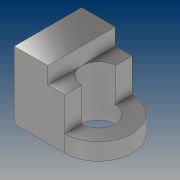
# Autodesk Inventor part: 34
Saved by Autodesk Inventor 2020.2 (Build 242310000, 310)
## iProperties
Created: 2020-09-17
Part Number: 34
Material: 鋼、碳鋼
Document SubType Name: Modeling
Designer: user
Density: 7.85 g/cm^3
Appearance: 半拋光
Mass: 345.4 g
Surface Area: 95.1327 cm^2
Volume: 44 cm^3
Author: user
Autodesk Inventor part; units mm, degrees
ref_plane "YZ Plane" through (0, 0, 0) normal (1, 0, 0) x (0, 1, 0)
ref_plane "XZ Plane" through (0, 0, 0) normal (0, 1, 0) x (-1, 0, 0)
ref_plane "XY Plane" through (0, 0, 0) normal (0, 0, 1) x (1, 0, 0)
sketch "草圖1" plane through (0, 0, 0) normal (0, 1, 0) x (-1, 0, 0)
  circle A0 centre (0, 0) radius 20
  line L0 (0, -20) -> (30, -20)
  line L1 (30, -20) -> (30, 20)
  line L2 (30, 20) -> (0, 20)
  line L3 (0, 20) -> (0, -20)
  point P0 (0, 20)
  dimension "d0" = 40
  dimension "d1" = 30
  constraints: 8 end point, 3 horizontal, 2 parallel, 1 coincident, 1 perpendicular, 3 other
  measures "d1" distance of L1.end L2.end
extrude "擠出1" add sketch "草圖1" along normal blind 40
sketch "草圖2" plane through (0, 40, 0) normal (0, 1, 0) x (1, 0, 0)
  line L0 (-30, 20) -> (0, 20) projected
  arc A0 (0, -20) -> (0, 20) centre (0, 0) ccw projected
  line L1 (0, -20) -> (-30, -20) projected
  line L2 (-30, -20) -> (-30, 20) projected
  line L3 (0, 27.0691) -> (-10, 27.0691)
  line L4 (-10, 27.0691) -> (-10, -29.9758)
  line L5 (-10, -29.9758) -> (0, -29.9758)
  line L6 (0, -29.9758) -> (0, 27.0691)
  dimension "d4" = 20
  dimension "d5" = 10
  constraints: 8 end point, 2 parallel, 1 horizontal, 1 perpendicular
  measures "d4" distance between parallel lines of L4 L2
  measures "d5" distance of L3.start L3.end
extrude "擠出2" cut sketch "草圖2" against normal blind 10 contours L4 L3 L6 L0 | L0 L6 L1 L4 | L1 L6 L5 L4
sketch "草圖3" plane through (0, 40, 0) normal (0, 1, 0) x (1, 0, 0)
  line L0 (0, -20) -> (0, 20) projected
  arc A0 (0, -20) -> (0, 20) centre (0, 0) ccw projected
  line L1 (-10, 20) -> (-10, -20) projected
  line L2 (-10, -20) -> (-30, -20) projected
  line L3 (-30, -20) -> (-30, 20) projected
  line L4 (-30, 20) -> (-10, 20) projected
  line L5 (0, -34.6108) -> (30.5971, -34.6108)
  line L6 (30.5971, -34.6108) -> (30.5971, 28.6775)
  line L7 (30.5971, 28.6775) -> (0, 28.6775)
  line L8 (0, 28.6775) -> (0, -34.6108)
  line L9 (0, 20) -> (0, -20) projected
  constraints: 8 end point, 2 parallel, 1 collinear, 1 horizontal, 1 perpendicular
extrude "擠出3" cut sketch "草圖3" against normal blind 30 contours L0 A0 | A0 L8 L7 L6 L5
sketch "草圖4" plane through (0, 0, 0) normal (0, -1, 0) x (1, 0, 0)
  arc A0 (0, -20) -> (0, 20) centre (0, 0) ccw projected
  constraints: 1 coincident
hole "孔1" at (0, 0, 0) direction (0, 1, 0) diameter 20 end through all
